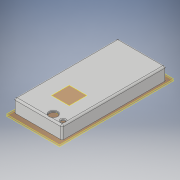
# Autodesk Inventor part: Pièce6
Saved by Autodesk Inventor 2019 (Build 230136000, 136)
## iProperties
Created: 2018-04-24
Part Number: Pièce6
Material: Générique
Document SubType Name: Modeling
Designer: Noah
Density: 1 g/cm^3
Appearance: Par défaut
Author: Noah
Autodesk Inventor part; units mm, degrees
ref_plane "YZ Plane" through (0, 0, 0) normal (1, 0, 0) x (0, 1, 0)
ref_plane "XZ Plane" through (0, 0, 0) normal (0, 1, 0) x (-1, 0, 0)
ref_plane "XY Plane" through (0, 0, 0) normal (0, 0, 1) x (1, 0, 0)
ref_plane "Plan de construction3" through (0, 20, 0) normal (0, 1, 0) x (1, 0, 0)
sketch "Esquisse7" plane through (0, 20, 0) normal (0, 1, 0) x (1, 0, 0)
  line L0 (-31.9796, 92.3061) -> (-31.9796, -36.6939) projected
  line L1 (28.0204, 92.3061) -> (-31.9796, 92.3061) projected
  line L2 (-31.9796, -36.6939) -> (28.0204, -36.6939)
  line L3 (28.0204, -36.6939) -> (28.0204, 92.3061)
  line L4 (28.0204, 92.3061) -> (-31.9796, 92.3061)
  line L5 (-31.9796, 92.3061) -> (-31.9796, -36.6939)
  line L6 (26.0204, 90.3061) -> (-29.9796, 90.3061) projected
  line L7 (26.0204, 90.3061) -> (26.0204, -34.6939) projected
  line L8 (-29.9796, 90.3061) -> (26.0204, 90.3061)
  line L9 (26.0204, 90.3061) -> (26.0204, -34.6939)
  line L10 (26.0204, -34.6939) -> (-29.9796, -34.6939)
  line L11 (-29.9796, -34.6939) -> (-29.9796, 90.3061)
  point P0 (0, 0)
  point P1 (6.0204, 92.3061)
  constraints: 16 end point, 4 parallel, 2 horizontal, 2 perpendicular
extrude "Extrusion6" add sketch "Esquisse7" along normal blind 14
ref_plane "Plan de construction4" through (0, 34, 0) normal (0, 1, 0) x (1, 0, 0)
sketch "Esquisse8" plane through (0, 34, 0) normal (0, 1, 0) x (1, 0, 0)
  line L0 (-31.9796, 92.3061) -> (-31.9796, -36.6939) projected
  line L1 (28.0204, -36.6939) -> (28.0204, 92.3061) projected
  line L2 (-31.9796, -36.6939) -> (28.0204, -36.6939)
  line L3 (28.0204, -36.6939) -> (28.0204, 92.3061)
  line L4 (28.0204, 92.3061) -> (-31.9796, 92.3061)
  line L5 (-31.9796, 92.3061) -> (-31.9796, -36.6939)
  point P0 (0, 0)
  constraints: 8 end point, 2 parallel, 1 horizontal, 1 perpendicular
extrude "Extrusion8" add sketch "Esquisse8" along normal blind 2
ref_plane "Plan de construction6" through (0, 36, 0) normal (0, 1, 0) x (1, 0, 0)
sketch "Esquisse9" plane through (0, 36, 0) normal (0, 1, 0) x (1, 0, 0)
  circle A0 centre (10.0204, -29.6939) radius 5
  line L0 (28.0204, -36.6939) -> (28.0204, 92.3061) projected
  line L1 (-31.9796, -36.6939) -> (28.0204, -36.6939) projected
  point P0 (0, 0)
  dimension "d75" = 10
  dimension "d76" = 18
  dimension "d77" = 7
  constraints: 1 centre point
  measures "d75" diameter of A0
  measures "d76" distance from line of L0 A0.centre
  measures "d77" distance from line of L1 A0.centre
extrude "Extrusion9" cut sketch "Esquisse9" against normal blind 3
ref_plane "Plan de construction5" through (0, 36, 0) normal (0, 1, 0) x (1, 0, 0)
sketch "Esquisse10" plane through (0, 36, 0) normal (0, 1, 0) x (1, 0, 0)
  circle A0 centre (23.0204, -30.6939) radius 2.5
  circle A1 centre (10.0204, -29.6939) radius 5 projected
  line L0 (-31.9796, -36.6939) -> (28.0204, -36.6939) projected
  point P0 (0, 0)
  dimension "d80" = 13
  dimension "d81" = 5
  dimension "d82" = 6
  constraints: 1 centre point
  measures "d80" horizontal distance of A1.centre A0.centre
  measures "d81" diameter of A0
  measures "d82" distance from line of L0 A0.centre
extrude "Extrusion10" cut sketch "Esquisse10" against normal blind 3 contours A0
ref_plane "Plan de construction1" through (0, 18, 0) normal (0, 1, 0) x (1, 0, 0)
ref_plane "Plan de construction2" through (0, 20, 0) normal (0, 1, 0) x (1, 0, 0)
fillet "Congé6" radius 2 8 edges at (28.0204, 36, -27.8061) (28.0204, 28, -92.3061) (28.0204, 28, 36.6939) (-31.9796, 28, -92.3061) (-1.9796, 36, -92.3061) (-31.9796, 36, -27.8061) (-1.9796, 36, 36.6939) (-31.9796, 28, 36.6939)
fillet "Congé7" radius 1 1 edges at (20.5204, 36, 30.6939)
fillet "Congé8" radius 0.5 1 edges at (5.0204, 36, 29.6939)
